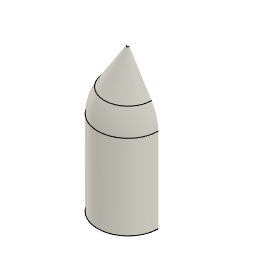
Razzetto 3 v2 (Autodesk Fusion 360 design; units mm, degrees)
Autodesk Fusion 360 part; units mm, degrees
note: some values were not read from the file. Set by a fixed rule: which sketch regions a step uses.
sketch "Schizzo2" plane through (0, 0, 0) normal (0, 1, 0) x (1, 0, 0)
  line L0 (6.25, 0) -> (6.25, -17.4188)
  line L1 (0.2968, -29.5251) -> (4.882, -22.1888)
  line L2 (0, -26.2264) -> (0, -29.6896)
  arc A0 (4.882, -22.1888) -> (6.25, -17.4188) centre (-2.75, -17.4188) ccw
  line L3 (0.9375, -28.5) -> (0, -28.5) construction
  arc A1 (0, -29.6896) -> (0.2968, -29.5251) centre (0, -29.3396) ccw
  line L4 (0, -26.2264) -> (3.186, -21.1288)
  arc A2 (3.186, -21.1288) -> (4.25, -17.4188) centre (-2.75, -17.4188) ccw
  line L5 (4.25, 0) -> (4.25, -17.4188)
  line L6 (6.25, 0) -> (4.25, 0)
  dimension "d9" = 6.25
  dimension "d24" = 9
  dimension "d25" = 0.35
  constraint tangent L1 A0
  constraint tangent L0 A0
  constraint horizontal L3
  constraint coincident L1 L3.start
  constraint coincident L2 L3.end
  constraint tangent L1 A1
  constraint concentric A0 A2
  constraint tangent L4 A2
  constraint tangent A2 L5
  constraint perpendicular L0 L6
  measures "d9" distance of origin L0.start
  measures "d24" radius of A0
  measures "d25" radius of A1
revolve "Rivoluzione6" add sketch "Schizzo2" angle 360 about axis through (0, 0, 26.2264) along (0, 0, 1)
revolve "Rivoluzione5" [suppressed]
revolve "Rivoluzione3" [suppressed]
ref_plane "Piano di lavoro1" through (0, -3, 0) normal (0, 1, 0) x (0, 0, 1)
revolve "Rivoluzione4" [suppressed]
revolve "Rivoluzione2" [suppressed]
sketch "Schizzo3" plane through (0, 0, 0) normal (0, 1, 0) x (1, 0, 0)
  line L0 (0, 1) -> (0, -23)
  constraint vertical L0
revolve "Rivoluzione1" [suppressed]
equation "d9 = ( 12.5 / 2 ) * 1 mm"
named bodies: "razzo", "fiammifero"
